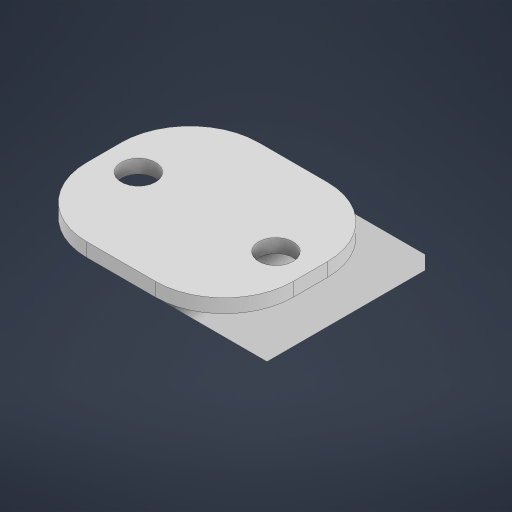
# Autodesk Inventor part: ancla
Saved by Autodesk Inventor 2023 (Build 270158000, 158)
## iProperties
Created: 2022-08-23
Part Number: ancla
Material: Generic
Document SubType Name: Modeling
Designer: marat
Density: 1 g/cm^3
Appearance: Default
Author: marat
Autodesk Inventor part; units mm, degrees
ref_plane "YZ Plane" through (0, 0, 0) normal (1, 0, 0) x (0, 1, 0)
ref_plane "XZ Plane" through (0, 0, 0) normal (0, 1, 0) x (-1, 0, 0)
ref_plane "XY Plane" through (0, 0, 0) normal (0, 0, 1) x (1, 0, 0)
sketch "Sketch1" plane through (0, 0, 0) normal (0, 1, 0) x (-1, 0, 0)
  line L0 (5, 12.5) -> (-5, 12.5)
  line L1 (-5, 12.5) -> (-5, -12.5)
  line L2 (-5, -12.5) -> (5, -12.5)
  line L3 (5, -12.5) -> (5, 12.5)
  line L4 (5, 12.5) -> (-5, -12.5) construction
  line L5 (-5, 12.5) -> (5, -12.5) construction
  line L6 (0, 7.5) -> (0, -7.5) construction
  line L7 (-1.5875, 7.5) -> (-1.5875, -7.5)
  line L8 (1.5875, -7.5) -> (1.5875, 7.5)
  arc A0 (1.5875, 7.5) -> (-1.5875, 7.5) centre (0, 7.5) ccw
  arc A1 (-1.5875, -7.5) -> (1.5875, -7.5) centre (0, -7.5) ccw
  point P0 (0, 0)
  point P1 (0, 0)
  dimension "d0" = 10
  dimension "d1" = 25
  dimension "d2" = 7.5
  dimension "d3" = 7.5
  dimension "d4" = 3.175
  constraints: 20 end point, 4 point on circle, 4 tangent, 3 midpoint, 3 parallel, 2 centre point, 1 horizontal, 1 perpendicular, 1 vertical
  measures "d0" distance of L2.end L1.end
  measures "d1" distance of L1.end L0.end
  measures "d2" distance of point (0, 0) L6.end
  measures "d3" distance of point (0, 0) L6.start
  measures "d4" diameter of A1
extrude "Extrusion1" add sketch "Sketch1" along normal blind 2
sketch "Sketch2" plane through (0, 2, 0) normal (0, 1, 0) x (1, 0, 0)
  line L0 (5, -12.5) -> (5, 12.5) projected
  line L1 (5, 12.5) -> (-5, 12.5) projected
  line L2 (-5, 12.5) -> (-5, -12.5) projected
  line L3 (-5, -12.5) -> (5, -12.5) projected
  arc A0 (-1.5875, -7.5) -> (1.5875, -7.5) centre (0, -7.5) ccw projected
  line L4 (-1.5875, -7.5) -> (-1.5875, 7.5) projected
  arc A1 (1.5875, 7.5) -> (-1.5875, 7.5) centre (0, 7.5) ccw projected
  line L5 (1.5875, 7.5) -> (1.5875, -7.5) projected
  line L6 (-3, -10.5) -> (-3, 10.5)
  line L7 (3, 10.5) -> (3, -10.5)
  line L8 (3, -10.5) -> (-3, -10.5)
  line L9 (-3, 10.5) -> (-3, 12.5)
  line L10 (3, 10.5) -> (3, 12.5)
  point P0 (0, 0)
  dimension "d7" = 2
  constraints: 10 end point, 2 perpendicular, 2 point on line, 1 other
  measures "d7" distance between parallel lines of L2 L6
sketch "Sketch3" plane through (0, 0, 0) normal (1, 0, 0) x (0, 1, 0)
  line L0 (2, 12.5) -> (16.2024, 26.7024)
  point P0 (0, 0)
  dimension "d15" = 20.0852
  constraints: 2 end point
  measures "d15" distance of L0.start L0.end
sweep "Sweep1" add profiles "Sketch2" path "Sketch3" contours L3 L2 L1 L9 L6 L8 L7 L10 L0
chamfer "Chamfer1" distance 2 angle 45 1 edges at (0, 0, 12.5)
sketch "Sketch5" plane through (-5, 16.2024, 26.7024) normal (0, 1, 0) x (1, 0, 0)
  line L0 (20, 0) -> (-10, 0)
  line L1 (-10, 0) -> (-10, 25)
  line L2 (-10, 25) -> (20, 25)
  line L3 (20, 25) -> (20, 0)
  line L4 (10, 0) -> (10, 25) projected
  circle A0 centre (15, 12.5) radius 2.5
  circle A1 centre (-5, 12.5) radius 2.5
  point P0 (5, 26.7024)
  dimension "d23" = 25
  dimension "d24" = 30
  dimension "d25" = 10
  dimension "d26" = 5
  dimension "d27" = 5
  dimension "d28" = 5
  dimension "d29" = 5
  constraints: 8 end point, 2 centre point, 2 parallel, 1 horizontal, 1 perpendicular
  measures "d23" distance of L0.end L1.end
  measures "d24" distance between parallel lines of L1 L3
  measures "d25" distance between parallel lines of L4 L3
  measures "d26" diameter of A0
  measures "d27" diameter of A1
  measures "d28" distance from line of L4 A0.centre
  measures "d29" distance from line of L1 A1.centre
extrude "Extrusion4" add sketch "Sketch5" along normal blind 2
fillet "Fillet1" radius 10 4 edges at (15, 17.2024, 1.7024) (-15, 17.2024, 1.7024) (-15, 17.2024, 26.7024) (15, 17.2024, 26.7024)
body "Solid1"
